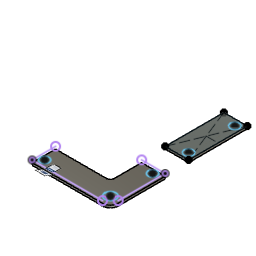
ScreenStabilizer (Autodesk Fusion 360 design; units mm, degrees)
Autodesk Fusion 360 part; units mm, degrees
sketch "Sketch1" plane through (0, 0, 0) normal (0, 0, 1) x (1, 0, 0)
  line L0 (0, 0) -> (100, 0)
  line L1 (100, 0) -> (100, 70)
  line L2 (100, 70) -> (70, 70)
  line L3 (70, 70) -> (70, 30)
  line L4 (70, 30) -> (0, 30)
  line L5 (0, 30) -> (0, 0)
  line L6 (-25, 0) -> (-25, 55) construction
  dimension "d1" = 30
  dimension "d2" = 30
  dimension "d3" = 100
  dimension "d4" = 70
  constraint coincident L0.start L5.end
  constraint horizontal L0
  constraint perpendicular L0 L1
  constraint perpendicular L1 L2
  constraint perpendicular L2 L3
  constraint perpendicular L3 L4
  constraint perpendicular L0 L5
  constraint vertical L6
  measures "d1" distance of L4.end L0.start
  measures "d2" distance of L1.end L2.end
  measures "d3" distance of L0.start L0.end
  measures "d4" distance of L0.end L1.end
extrude "Extrude1" add sketch "Sketch1" along normal blind 3 makes body 1
ref_plane "WorkPlane1" through (-30, 0, 0) normal (1, 0, 0) x (0, 1, 0)
sketch "Sketch2" plane through (0, 0, 3) normal (0, 0, 1) x (-1, 0, 0)
  line L0 (0, -30) -> (0, 0)
  line L1 (0, 0) -> (-100, 0)
  line L2 (-100, 0) -> (-100, -70)
  line L3 (-100, -70) -> (-70, -70)
  line L4 (-70, -70) -> (-70, -30)
  line L5 (-70, -30) -> (0, -30)
  line L6 (-100, -100) -> (-70, -100)
  line L7 (-70, -100) -> (-70, -175)
  line L8 (-70, -175) -> (-100, -175)
  line L9 (-100, -175) -> (-100, -100)
  dimension "d10" = 30
  dimension "d11" = 75
  constraint horizontal L6
  constraint perpendicular L6 L7
  constraint perpendicular L7 L8
  constraint perpendicular L6 L9
  measures "d10" distance of L7.end L8.end
  measures "d11" distance of L6.end L7.end
extrude "Extrude2" add sketch "Sketch2" along normal blind 3 separate body contours L6 L7 L8 L9 makes body 2
fillet "Fillet1" radius 10 1 edges at (100, 0, 1.5) on bodies 1
fillet "Fillet2" radius 5 1 edges at (70, 30, 1.5) on bodies 1
sketch "Sketch3" plane through (0, 0, 6) normal (0, 0, 1) x (-1, 0, 0)
  line L0 (-100, -175) -> (-70, -175)
  line L1 (-70, -175) -> (-70, -100)
  line L2 (-70, -100) -> (-100, -100)
  line L3 (-100, -100) -> (-100, -175)
  circle A0 centre (-92, -108) radius 5.6569
  line L4 (-70, -175) -> (-100, -100) construction
  line L5 (-70, -100) -> (-100, -175) construction
  line L6 (-85, -137.5) -> (-100, -137.5) construction
  circle A1 centre (-90, -10) radius 7.0711
  circle A2 centre (-92, -62) radius 5.6189
  circle A3 centre (-8, -8) radius 5.5698
  line L7 (-100, -10) -> (-100, -70)
  line L8 (-100, -70) -> (-70, -70)
  line L9 (0, 0) -> (-90, 0)
  line L10 (0, -30) -> (0, 0)
  circle A4 centre (-92, -167) radius 5.6569
  dimension "d18" = 8
  dimension "d19" = 8
  dimension "d20" = 8
  dimension "d21" = 8
  dimension "d22" = 10
  dimension "d23" = 10
  dimension "d24" = 8
  dimension "d25" = 8
  constraint coincident L0.end L1.start
  constraint coincident L2.end L3.start
  constraint coincident L1.end L2.start
  constraint coincident L0.start L3.end
  constraint midpoint L4 L6.start
  constraint midpoint L3 L6.end
  constraint symmetric A0 L6 A4
  measures "d18" distance of L3 A0.centre
  measures "d19" distance of L2 A0.centre
  measures "d20" distance of A2.centre L7
  measures "d21" distance of A2.centre L8
  measures "d22" distance of A1.centre L7
  measures "d23" distance of A1.centre L9
  measures "d24" distance of A3.centre L10
  measures "d25" distance of A3.centre L9
